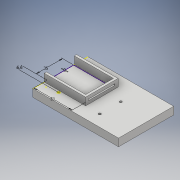
# Autodesk Inventor part: Back Plate test03
Saved by Autodesk Inventor 2018 (Build 220112000, 112)
## iProperties
Created: 2022-01-10
Part Number: Back Plate test03
Material: Generic
Document SubType Name: Modeling
Designer: Stewart Alexander
Density: 1 g/cm^3
Appearance: Default
Author: Stewart Alexander
Autodesk Inventor part; units mm, degrees
ref_plane "YZ Plane" through (0, 0, 0) normal (1, 0, 0) x (0, 1, 0)
ref_plane "XZ Plane" through (0, 0, 0) normal (0, 1, 0) x (-1, 0, 0)
ref_plane "XY Plane" through (0, 0, 0) normal (0, 0, 1) x (1, 0, 0)
sketch "Arduino Uno" plane through (0, 0, 0) normal (0, 0, 1) x (1, 0, 0)
  line L0 (0, 0) -> (68.6, 0)
  line L1 (68.6, 0) -> (68.6, 53.3)
  line L2 (68.6, 53.3) -> (0, 53.3)
  line L3 (0, 53.3) -> (0, 0)
  circle A0 centre (14, 2.5) radius 1.6
  circle A1 centre (15.3, 50.7) radius 1.6
  circle A2 centre (66.1, 5.1) radius 1.6
  circle A3 centre (66.1, 33) radius 1.6
  dimension "d6" = 68.6
  dimension "d7" = 53.3
  dimension "d8" = 3.2
  dimension "d12" = 14
  dimension "d13" = 2.5
  dimension "d14" = 3.2
  dimension "d15" = 1.3
  dimension "d16" = 3.2
  dimension "d18" = 2.5
  dimension "d19" = 5.1
  dimension "d20" = 3.2
  dimension "d21" = 27.9
  dimension "d22" = 2.5
  dimension "d26" = 2.6
  constraints: 8 end point, 4 centre point, 2 parallel, 1 horizontal, 1 perpendicular
  measures "d6" distance of L2.end L1.end
  measures "d7" distance of L0.end L1.end
  measures "d8" diameter of A0
  measures "d12" distance from line of L3 A0.centre
  measures "d13" distance from line of L0 A0.centre
  measures "d14" diameter of A1
  measures "d15" horizontal distance of A0.centre A1.centre
  measures "d16" diameter of A2
  measures "d18" distance from line of L1 A2.centre
  measures "d19" distance from line of L0 A2.centre
  measures "d20" diameter of A3
  measures "d21" distance of A2.centre A3.centre
  measures "d22" distance from line of L1 A3.centre
  measures "d26" distance from line of L2 A1.centre
sketch "Sketch2" plane through (0, 0, 0) normal (0, 0, 1) x (1, 0, 0)
  line L0 (-7.6136, -10.2044) -> (-7.6136, 63.0956)
  line L1 (-7.6136, 63.0956) -> (106.3864, 63.0956)
  line L2 (106.3864, 63.0956) -> (106.3864, -10.2044)
  line L3 (106.3864, -10.2044) -> (-7.6136, -10.2044)
  dimension "d29" = 114
  dimension "d39" = 73.3
  constraints: 8 end point, 3 perpendicular
  measures "d29" distance of L0.end L1.end
  measures "d39" distance of L0.start L0.end
extrude "Back Plate" add sketch "Sketch2" against normal blind 10
extrude "Uno Mounting Holes" cut sketch "Arduino Uno" against normal blind 5 contours A0 | A1 | A2 | A3
sketch "3.5\" TFT LCD Screen" plane through (0, 0, 0) normal (0, 0, 1) x (1, 0, 0)
  line L0 (88.6005, 0.0003) -> (88.6005, 53.3003)
  line L1 (88.6005, 53.3003) -> (10.6005, 53.3003)
  line L2 (10.6005, 53.3003) -> (10.6005, 0.0003)
  line L3 (10.6005, 0.0003) -> (88.6005, 0.0003)
  circle A0 centre (66.1, 5.1) radius 1.6 projected
  circle A1 centre (14, 2.5) radius 1.6 projected
  circle A2 centre (15.3, 50.7) radius 1.6 projected
  circle A3 centre (66.1, 33) radius 1.6 projected
  line L4 (-7.6136, -10.2044) -> (-7.6136, 63.0956) projected
  line L5 (106.3864, -10.2044) -> (-7.6136, -10.2044) projected
  line L6 (106.3864, 63.0956) -> (106.3864, -10.2044) projected
  line L7 (-7.6136, 63.0956) -> (106.3864, 63.0956) projected
  point P0 (0, 0)
  point P1 (68.6, 0)
  dimension "d35" = 78
  dimension "d36" = 53.3
  dimension "d37" = 78
  dimension "d38" = 53.3
  constraints: 8 end point
  measures "d35" distance of L2.end L0.start
  measures "d36" distance of L1.end L2.end
  measures "d37" distance of L0.end L1.end
  measures "d38" distance of L0.start L0.end
sketch "SD Card Slot" plane through (0, 0, 0) normal (0, 0, 1) x (1, 0, 0)
  line L0 (43.3864, 9.1) -> (-7.6136, 9.1)
  line L1 (-7.6136, 9.1) -> (-7.6136, 44.1)
  line L2 (-7.6136, 44.1) -> (43.3864, 44.1)
  line L3 (43.3864, 44.1) -> (43.3864, 9.1)
  circle A0 centre (14, 2.5) radius 1.6 projected
  line L4 (-7.6136, -10.2044) -> (-7.6136, 63.0956) projected
  circle A1 centre (15.3, 50.7) radius 1.6 projected
  point P0 (0, 0)
  dimension "d41" = 35
  dimension "d42" = 51
  dimension "d44" = 6.6
  dimension "d45" = 0
  constraints: 8 end point, 2 parallel, 1 horizontal, 1 perpendicular
  measures "d41" distance of L0.end L1.end
  measures "d42" distance of L0.start L0.end
  measures "d44" distance from line of L0 A0.centre
  measures "d45" distance between parallel lines of L4 L1
sketch "Sketch5" plane through (0, 0, 0) normal (0, 0, 1) x (1, 0, 0)
  line L0 (43.3864, 9.1) -> (-7.6136, 9.1) projected
  line L1 (43.3864, 44.1) -> (43.3864, 9.1) projected
  line L2 (-7.6136, 44.1) -> (43.3864, 44.1) projected
  line L3 (-7.6136, 9.1) -> (-7.6136, 44.1) projected
  line L4 (44.3864, 8.1) -> (44.3864, 45.1)
  line L5 (44.3864, 8.1) -> (-7.6136, 8.1)
  line L6 (-7.6136, -10.2044) -> (-7.6136, 63.0956) projected
  line L7 (44.3864, 45.1) -> (-7.6136, 45.1)
  line L8 (-7.6136, 45.1) -> (-7.6136, 48.1)
  line L9 (-7.6136, 48.1) -> (47.3864, 48.1)
  line L10 (-7.6136, 8.1) -> (-7.6136, 5.1)
  line L11 (-7.6136, 5.1) -> (47.3864, 5.1)
  line L12 (47.3864, 5.1) -> (47.3864, 48.1)
  point P0 (0, 0)
  dimension "d47" = 3
  dimension "d48" = 55
  dimension "d49" = 3
  constraints: 16 end point, 4 perpendicular, 3 point on line, 1 horizontal, 1 parallel
  measures "d47" distance of L7.end L8.end
  measures "d48" distance of L8.end L9.end
  measures "d49" distance of L5.end L10.end
extrude "SD Card Slot Slot" add sketch "Sketch5" along normal blind 10 contours L5 L4 L7 L6 L9 L12 L11
sketch "Sketch6" plane through (47.3864, 5.1, 0) normal (1, 0, 0) x (0, 0, -1)
  line L0 (0, 43) -> (0, 0) projected
  line L1 (0, 43) -> (-10, 43) projected
  line L2 (-10, 0) -> (-10, 43) projected
  line L3 (0, 0) -> (-10, 0) projected
  line L4 (-6, 39) -> (-4, 39)
  line L5 (-4, 39) -> (-4, 4)
  line L6 (-4, 4) -> (-6, 4)
  line L7 (-6, 4) -> (-6, 39)
  point P0 (0, -5.1)
  dimension "d52" = 4
  constraints: 8 end point, 3 other
  measures "d52" distance between parallel lines of L2 L7
extrude "SD Ribbon Slot" cut sketch "Sketch6" against normal through all contours L4 L5 L6 L7
body "Solid1"
